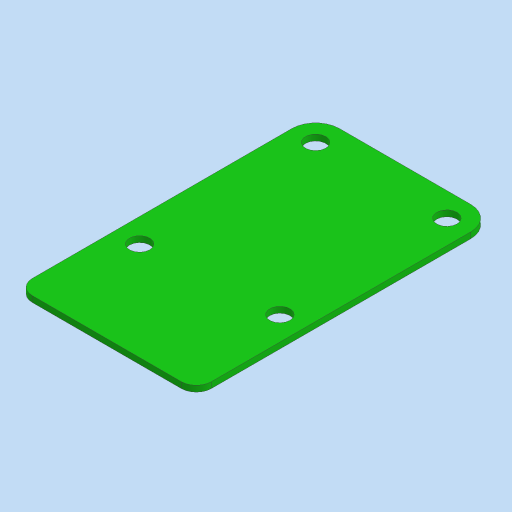
# Autodesk Inventor part: mcu_pcb
Saved by Autodesk Inventor 2024 (Build 280153000, 153)
## iProperties
Created: 2025-05-06
Part Number: mcu_pcb
Material: Generic
Document SubType Name: Modeling
Designer: XxPan
Density: 1 g/cm^3
Appearance: Default
Author: XxPan
Autodesk Inventor part; units mm, degrees
ref_plane "YZ Plane" through (0, 0, 0) normal (1, 0, 0) x (0, 1, 0)
ref_plane "XZ Plane" through (0, 0, 0) normal (0, 1, 0) x (-1, 0, 0)
ref_plane "XY Plane" through (0, 0, 0) normal (0, 0, 1) x (1, 0, 0)
sketch "Sketch1" plane through (0, 0, 0) normal (0, 1, 0) x (-1, 0, 0)
  line L0 (15, 25) -> (-15, 25)
  line L1 (-15, 25) -> (-15, -25)
  line L2 (-15, -25) -> (15, -25)
  line L3 (15, -25) -> (15, 25)
  line L4 (21, 0) -> (-21, 0) construction
  line L5 (0, -35) -> (0, 35) construction
  point P0 (0, 0)
  dimension "d11" = 15
  dimension "d12" = 15
  dimension "d13" = 25
  dimension "d14" = 25
  constraints: 8 end point, 2 parallel, 1 horizontal, 1 perpendicular
  measures "d11" distance between parallel lines of L1 L5
  measures "d12" distance between parallel lines of L5 L3
  measures "d13" distance between parallel lines of L4 L0
  measures "d14" distance between parallel lines of L4 L2
extrude "Extrusion1" add sketch "Sketch1" against normal blind 1
fillet "Fillet1" radius 2.5 2 edges at (-15, -0.5, 25) (15, -0.5, 25)
fillet "Fillet2" radius 4 2 edges at (-15, -0.5, -25) (15, -0.5, -25)
sketch "Sketch3" plane through (0, 0, 0) normal (0, 1, 0) x (1, 0, 0)
  arc A0 (15, 21) -> (11, 25) centre (11, 21) ccw projected
  arc A1 (-11, 25) -> (-15, 21) centre (-11, 21) ccw projected
  line L0 (15, -22.5) -> (15, 21) projected
  line L1 (-15, 21) -> (-15, -22.5) projected
  line L2 (-12.5, -25) -> (12.5, -25) projected
  point P0 (0, 0)
  point P1 (11, -7)
  point P2 (-11, -8.5)
  point P3 (12.5, -25)
  dimension "d24" = 4
  dimension "d25" = 4
  dimension "d52" = 18
  dimension "d53" = 1.5
  constraints: 2 coincident, 1 other
  measures "d24" distance from line of L0 point (11, -7)
  measures "d25" distance from line of L1 point (-11, -8.5)
  measures "d53" vertical distance of point (-11, -8.5) point (11, -7)
hole "Hole2" at (-11, 0, -21) at (11, 0, -21) at (11, 0, 7) at (-11, 0, 8.5) direction (0, -1, 0) diameter 3.4 end through all
body "Solid1"
